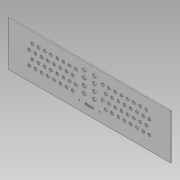
# Autodesk Inventor part: FrontPanel
Saved by Autodesk Inventor 2021.4 (Build 254397000, 397)
## iProperties
Created: 2022-05-18
Part Number: FrontPanel
Material: Generic
Document SubType Name: Modeling
Designer: LaborAdmin
Density: 1 g/cm^3
Appearance: Default
Author: LaborAdmin
Autodesk Inventor part; units mm, degrees
ref_plane "YZ Plane" through (0, 0, 0) normal (1, 0, 0) x (0, 1, 0)
ref_plane "XZ Plane" through (0, 0, 0) normal (0, 1, 0) x (-1, 0, 0)
ref_plane "XY Plane" through (0, 0, 0) normal (0, 0, 1) x (1, 0, 0)
sketch "Sketch1" plane through (0, 0, 0) normal (0, 0, 1) x (1, 0, 0)
  line L0 (-241, 66.5) -> (241, 66.5)
  line L1 (241, 66.5) -> (241, -66.5)
  line L2 (241, -66.5) -> (-241, -66.5)
  line L3 (-241, -66.5) -> (-241, 66.5)
  line L4 (-241, 66.5) -> (241, -66.5) construction
  line L5 (241, 66.5) -> (-241, -66.5) construction
  point P0 (0, 0)
  dimension "d0" = 482
  dimension "d1" = 133
  constraints: 12 end point, 2 midpoint, 2 parallel, 1 horizontal, 1 perpendicular
  measures "d0" distance of L1.end L2.end
  measures "d1" distance of L2.end L0.start
extrude "Extrusion1" add sketch "Sketch1" against normal blind 3
sketch "Sketch2" plane through (0, 0, 0) normal (0, 0, 1) x (1, 0, 0)
  line L0 (-197, -50) -> (197, -50) construction
  line L1 (197, -50) -> (197, 50) construction
  line L2 (197, 50) -> (-197, 50) construction
  line L3 (-197, 50) -> (-197, -50) construction
  line L4 (-197, -50) -> (197, 50) construction
  line L5 (197, -50) -> (-197, 50) construction
  line L6 (-241, 66.5) -> (241, 66.5) construction
  line L7 (0, 66.5) -> (0, -66.5) construction
  line L8 (241, -66.5) -> (-241, -66.5) construction
  line L9 (15, 66.5) -> (15, -66.5) construction
  arc A0 (11.9308, 48.89) -> (18.0692, 48.89) centre (15, 45) ccw
  line L10 (11.9308, 48.89) -> (18.0692, 48.89)
  arc A1 (11.9308, 28.89) -> (18.0692, 28.89) centre (15, 25) ccw
  line L11 (11.9308, 28.89) -> (18.0692, 28.89)
  arc A2 (11.9308, 8.89) -> (18.0692, 8.89) centre (15, 5) ccw
  line L12 (11.9308, 8.89) -> (18.0692, 8.89)
  arc A3 (11.9308, -11.11) -> (18.0692, -11.11) centre (15, -15) ccw
  line L13 (11.9308, -11.11) -> (18.0692, -11.11)
  arc A4 (-18.0692, 48.89) -> (-11.9308, 48.89) centre (-15, 45) ccw
  line L14 (-11.9308, 48.89) -> (-18.0692, 48.89)
  line L15 (-11.9308, 28.89) -> (-18.0692, 28.89)
  arc A5 (-18.0692, 28.89) -> (-11.9308, 28.89) centre (-15, 25) ccw
  line L16 (-11.9308, 8.89) -> (-18.0692, 8.89)
  arc A6 (-18.0692, 8.89) -> (-11.9308, 8.89) centre (-15, 5) ccw
  line L17 (-11.9308, -11.11) -> (-18.0692, -11.11)
  arc A7 (-18.0692, -11.11) -> (-11.9308, -11.11) centre (-15, -15) ccw
  point P0 (0, 0)
  dimension "d4" = 394
  dimension "d5" = 100
  dimension "d6" = 15
  dimension "d7" = 5
  dimension "dBNC" = 9.91
  dimension "hBNC" = 3.89
  dimension "d12" = 9.91
  dimension "d13" = 3.89
  dimension "d14" = 9.91
  dimension "d15" = 3.89
  dimension "d16" = 9.91
  dimension "d17" = 3.89
  dimension "distBNC" = 20
  dimension "d19" = 20
  dimension "d20" = 20
  constraints: 32 end point, 16 point on circle, 16 symmetric about line, 8 centre point, 8 coincident, 6 point on line, 5 horizontal, 4 midpoint, 2 parallel, 1 perpendicular, 1 vertical, 4 other
  measures "d4" distance of L1.end L2.end
  measures "d5" distance of L0.end L1.end
  measures "d6" distance between parallel lines of L7 L9
  measures "d7" distance from line of L2 point (15, 45)
  measures "dBNC" diameter of A0
  measures "hBNC" distance from line of L10 point (15, 45)
  measures "d12" diameter of A1
  measures "d13" distance from line of L11 point (15, 25)
  measures "d14" diameter of A2
  measures "d15" distance from line of L12 point (15, 5)
  measures "d16" diameter of A3
  measures "d17" distance from line of L13 point (15, -15)
  measures "distBNC" distance of point (15, 25) point (15, 45)
  measures "d19" distance of point (15, 5) A1.centre
  measures "d20" distance of point (15, -15) point (15, 5)
extrude "Extrusion2" cut sketch "Sketch2" against normal blind 3
sketch "Sketch3" plane through (0, 0, 0) normal (0, 0, 1) x (1, 0, 0)
  line L0 (-241, 66.5) -> (241, 66.5) projected
  line L1 (0, 66.5) -> (0, -66.5) construction
  line L2 (241, -66.5) -> (-241, -66.5) projected
  line L3 (-197, -50) -> (197, -50) construction
  line L4 (197, -50) -> (197, 50) construction
  line L5 (197, 50) -> (-197, 50) construction
  line L6 (-197, 50) -> (-197, -50) construction
  line L7 (-197, -50) -> (197, 50) construction
  line L8 (197, -50) -> (-197, 50) construction
  arc A0 (11.9308, 48.89) -> (18.0692, 48.89) centre (15, 45) ccw projected
  arc A1 (11.9308, 28.89) -> (18.0692, 28.89) centre (15, 25) ccw projected
  line L9 (15, 45) -> (15, 25) construction
  line L10 (15, 35) -> (197, 35) construction
  arc A2 (11.9308, 8.89) -> (18.0692, 8.89) centre (15, 5) ccw projected
  line L11 (15, 25) -> (15, 5) construction
  arc A3 (11.9308, -11.11) -> (18.0692, -11.11) centre (15, -15) ccw projected
  line L12 (15, 5) -> (15, -15) construction
  line L13 (15, 15) -> (197, 15) construction
  line L14 (15, -5) -> (197, -5) construction
  line L15 (15, -15) -> (15, -35) construction
  line L16 (15, -25) -> (197, -25) construction
  arc A4 (37.5917, 38.225) -> (42.4083, 38.225) centre (40, 35) ccw
  line L17 (37.5917, 38.225) -> (42.4083, 38.225)
  arc A5 (56.0917, 38.225) -> (60.9083, 38.225) centre (58.5, 35) ccw
  line L18 (56.0917, 38.225) -> (60.9083, 38.225)
  arc A6 (74.5917, 38.225) -> (79.4083, 38.225) centre (77, 35) ccw
  line L19 (74.5917, 38.225) -> (79.4083, 38.225)
  arc A7 (93.0917, 38.225) -> (97.9083, 38.225) centre (95.5, 35) ccw
  line L20 (93.0917, 38.225) -> (97.9083, 38.225)
  arc A8 (111.5917, 38.225) -> (116.4083, 38.225) centre (114, 35) ccw
  line L21 (111.5917, 38.225) -> (116.4083, 38.225)
  arc A9 (130.0917, 38.225) -> (134.9083, 38.225) centre (132.5, 35) ccw
  line L22 (130.0917, 38.225) -> (134.9083, 38.225)
  arc A10 (148.5917, 38.225) -> (153.4083, 38.225) centre (151, 35) ccw
  line L23 (148.5917, 38.225) -> (153.4083, 38.225)
  arc A11 (167.0917, 38.225) -> (171.9083, 38.225) centre (169.5, 35) ccw
  line L24 (167.0917, 38.225) -> (171.9083, 38.225)
  arc A12 (46.8417, 18.225) -> (51.6583, 18.225) centre (49.25, 15) ccw
  line L25 (46.8417, 18.225) -> (51.6583, 18.225)
  arc A13 (65.3417, 18.225) -> (70.1583, 18.225) centre (67.75, 15) ccw
  line L26 (65.3417, 18.225) -> (70.1583, 18.225)
  arc A14 (83.8417, 18.225) -> (88.6583, 18.225) centre (86.25, 15) ccw
  line L27 (83.8417, 18.225) -> (88.6583, 18.225)
  arc A15 (102.3417, 18.225) -> (107.1583, 18.225) centre (104.75, 15) ccw
  line L28 (102.3417, 18.225) -> (107.1583, 18.225)
  arc A16 (120.8417, 18.225) -> (125.6583, 18.225) centre (123.25, 15) ccw
  line L29 (120.8417, 18.225) -> (125.6583, 18.225)
  arc A17 (139.3417, 18.225) -> (144.1583, 18.225) centre (141.75, 15) ccw
  line L30 (139.3417, 18.225) -> (144.1583, 18.225)
  arc A18 (157.8417, 18.225) -> (162.6583, 18.225) centre (160.25, 15) ccw
  line L31 (157.8417, 18.225) -> (162.6583, 18.225)
  arc A19 (176.3417, 18.225) -> (181.1583, 18.225) centre (178.75, 15) ccw
  line L32 (176.3417, 18.225) -> (181.1583, 18.225)
  arc A20 (37.5917, -1.775) -> (42.4083, -1.775) centre (40, -5) ccw
  line L33 (37.5917, -1.775) -> (42.4083, -1.775)
  line L34 (56.0917, -1.775) -> (60.9083, -1.775)
  arc A21 (56.0917, -1.775) -> (60.9083, -1.775) centre (58.5, -5) ccw
  line L35 (74.5917, -1.775) -> (79.4083, -1.775)
  arc A22 (74.5917, -1.775) -> (79.4083, -1.775) centre (77, -5) ccw
  line L36 (93.0917, -1.775) -> (97.9083, -1.775)
  arc A23 (93.0917, -1.775) -> (97.9083, -1.775) centre (95.5, -5) ccw
  line L37 (111.5917, -1.775) -> (116.4083, -1.775)
  arc A24 (111.5917, -1.775) -> (116.4083, -1.775) centre (114, -5) ccw
  line L38 (130.0917, -1.775) -> (134.9083, -1.775)
  arc A25 (130.0917, -1.775) -> (134.9083, -1.775) centre (132.5, -5) ccw
  line L39 (148.5917, -1.775) -> (153.4083, -1.775)
  arc A26 (148.5917, -1.775) -> (153.4083, -1.775) centre (151, -5) ccw
  line L40 (167.0917, -1.775) -> (171.9083, -1.775)
  arc A27 (167.0917, -1.775) -> (171.9083, -1.775) centre (169.5, -5) ccw
  arc A28 (46.8417, -21.775) -> (51.6583, -21.775) centre (49.25, -25) ccw
  line L41 (46.8417, -21.775) -> (51.6583, -21.775)
  arc A29 (65.3417, -21.775) -> (70.1583, -21.775) centre (67.75, -25) ccw
  line L42 (65.3417, -21.775) -> (70.1583, -21.775)
  arc A30 (83.8417, -21.775) -> (88.6583, -21.775) centre (86.25, -25) ccw
  line L43 (83.8417, -21.775) -> (88.6583, -21.775)
  arc A31 (102.3417, -21.775) -> (107.1583, -21.775) centre (104.75, -25) ccw
  line L44 (102.3417, -21.775) -> (107.1583, -21.775)
  arc A32 (120.8417, -21.775) -> (125.6583, -21.775) centre (123.25, -25) ccw
  line L45 (120.8417, -21.775) -> (125.6583, -21.775)
  arc A33 (139.3417, -21.775) -> (144.1583, -21.775) centre (141.75, -25) ccw
  line L46 (139.3417, -21.775) -> (144.1583, -21.775)
  arc A34 (157.8417, -21.775) -> (162.6583, -21.775) centre (160.25, -25) ccw
  line L47 (157.8417, -21.775) -> (162.6583, -21.775)
  arc A35 (176.3417, -21.775) -> (181.1583, -21.775) centre (178.75, -25) ccw
  line L48 (176.3417, -21.775) -> (181.1583, -21.775)
  arc A36 (-42.4083, 38.225) -> (-37.5917, 38.225) centre (-40, 35) ccw
  line L49 (-37.5917, 38.225) -> (-42.4083, 38.225)
  line L50 (-56.0917, 38.225) -> (-60.9083, 38.225)
  arc A37 (-60.9083, 38.225) -> (-56.0917, 38.225) centre (-58.5, 35) ccw
  line L51 (-74.5917, 38.225) -> (-79.4083, 38.225)
  arc A38 (-79.4083, 38.225) -> (-74.5917, 38.225) centre (-77, 35) ccw
  line L52 (-93.0917, 38.225) -> (-97.9083, 38.225)
  arc A39 (-97.9083, 38.225) -> (-93.0917, 38.225) centre (-95.5, 35) ccw
  line L53 (-111.5917, 38.225) -> (-116.4083, 38.225)
  arc A40 (-116.4083, 38.225) -> (-111.5917, 38.225) centre (-114, 35) ccw
  line L54 (-130.0917, 38.225) -> (-134.9083, 38.225)
  arc A41 (-134.9083, 38.225) -> (-130.0917, 38.225) centre (-132.5, 35) ccw
  line L55 (-148.5917, 38.225) -> (-153.4083, 38.225)
  arc A42 (-153.4083, 38.225) -> (-148.5917, 38.225) centre (-151, 35) ccw
  line L56 (-167.0917, 38.225) -> (-171.9083, 38.225)
  arc A43 (-171.9083, 38.225) -> (-167.0917, 38.225) centre (-169.5, 35) ccw
  arc A44 (-51.6583, 18.225) -> (-46.8417, 18.225) centre (-49.25, 15) ccw
  line L57 (-46.8417, 18.225) -> (-51.6583, 18.225)
  arc A45 (-70.1583, 18.225) -> (-65.3417, 18.225) centre (-67.75, 15) ccw
  line L58 (-65.3417, 18.225) -> (-70.1583, 18.225)
  arc A46 (-88.6583, 18.225) -> (-83.8417, 18.225) centre (-86.25, 15) ccw
  line L59 (-83.8417, 18.225) -> (-88.6583, 18.225)
  arc A47 (-107.1583, 18.225) -> (-102.3417, 18.225) centre (-104.75, 15) ccw
  line L60 (-102.3417, 18.225) -> (-107.1583, 18.225)
  arc A48 (-125.6583, 18.225) -> (-120.8417, 18.225) centre (-123.25, 15) ccw
  line L61 (-120.8417, 18.225) -> (-125.6583, 18.225)
  arc A49 (-144.1583, 18.225) -> (-139.3417, 18.225) centre (-141.75, 15) ccw
  line L62 (-139.3417, 18.225) -> (-144.1583, 18.225)
  arc A50 (-162.6583, 18.225) -> (-157.8417, 18.225) centre (-160.25, 15) ccw
  line L63 (-157.8417, 18.225) -> (-162.6583, 18.225)
  arc A51 (-181.1583, 18.225) -> (-176.3417, 18.225) centre (-178.75, 15) ccw
  line L64 (-176.3417, 18.225) -> (-181.1583, 18.225)
  arc A52 (-42.4083, -1.775) -> (-37.5917, -1.775) centre (-40, -5) ccw
  line L65 (-74.5917, -1.775) -> (-79.4083, -1.775)
  line L66 (-83.8417, -21.775) -> (-88.6583, -21.775)
  line L67 (-65.3417, -21.775) -> (-70.1583, -21.775)
  arc A53 (-70.1583, -21.775) -> (-65.3417, -21.775) centre (-67.75, -25) ccw
  arc A54 (-88.6583, -21.775) -> (-83.8417, -21.775) centre (-86.25, -25) ccw
  line L68 (-102.3417, -21.775) -> (-107.1583, -21.775)
  arc A55 (-107.1583, -21.775) -> (-102.3417, -21.775) centre (-104.75, -25) ccw
  line L69 (-56.0917, -1.775) -> (-60.9083, -1.775)
  arc A56 (-60.9083, -1.775) -> (-56.0917, -1.775) centre (-58.5, -5) ccw
  arc A57 (-79.4083, -1.775) -> (-74.5917, -1.775) centre (-77, -5) ccw
  line L70 (-93.0917, -1.775) -> (-97.9083, -1.775)
  arc A58 (-97.9083, -1.775) -> (-93.0917, -1.775) centre (-95.5, -5) ccw
  line L71 (-130.0917, -1.775) -> (-134.9083, -1.775)
  arc A59 (-134.9083, -1.775) -> (-130.0917, -1.775) centre (-132.5, -5) ccw
  line L72 (-120.8417, -21.775) -> (-125.6583, -21.775)
  arc A60 (-125.6583, -21.775) -> (-120.8417, -21.775) centre (-123.25, -25) ccw
  line L73 (-111.5917, -1.775) -> (-116.4083, -1.775)
  arc A61 (-116.4083, -1.775) -> (-111.5917, -1.775) centre (-114, -5) ccw
  line L74 (-176.3417, -21.775) -> (-181.1583, -21.775)
  arc A62 (-181.1583, -21.775) -> (-176.3417, -21.775) centre (-178.75, -25) ccw
  arc A63 (-144.1583, -21.775) -> (-139.3417, -21.775) centre (-141.75, -25) ccw
  line L75 (-139.3417, -21.775) -> (-144.1583, -21.775)
  line L76 (-148.5917, -1.775) -> (-153.4083, -1.775)
  arc A64 (-153.4083, -1.775) -> (-148.5917, -1.775) centre (-151, -5) ccw
  arc A65 (-162.6583, -21.775) -> (-157.8417, -21.775) centre (-160.25, -25) ccw
  line L77 (-157.8417, -21.775) -> (-162.6583, -21.775)
  arc A66 (-171.9083, -1.775) -> (-167.0917, -1.775) centre (-169.5, -5) ccw
  line L78 (-167.0917, -1.775) -> (-171.9083, -1.775)
  line L79 (-37.5917, -1.775) -> (-42.4083, -1.775)
  line L80 (-46.8417, -21.775) -> (-51.6583, -21.775)
  arc A67 (-51.6583, -21.775) -> (-46.8417, -21.775) centre (-49.25, -25) ccw
  point P0 (0, 0)
  dimension "d23" = 394
  dimension "d24" = 100
  dimension "d25" = 20
  dimension "dXLR" = 8.05
  dimension "distBNC_XLR" = 25
  dimension "hXLR" = 7.25
  dimension "d29" = 8.05
  dimension "d30" = 7.25
  dimension "d31" = 8.05
  dimension "d32" = 7.25
  dimension "d33" = 8.05
  dimension "d34" = 7.25
  dimension "d35" = 8.05
  dimension "d36" = 7.25
  dimension "d37" = 8.05
  dimension "d38" = 7.25
  dimension "d39" = 8.05
  dimension "d40" = 7.25
  dimension "d41" = 8.05
  dimension "d42" = 7.25
  dimension "distXLR" = 18.5
  dimension "d44" = 18.5
  dimension "d45" = 18.5
  dimension "d46" = 18.5
  dimension "d47" = 18.5
  dimension "d48" = 18.5
  dimension "d49" = 18.5
  dimension "d50" = 8.05
  dimension "d73" = 34.25
  dimension "d74" = 7.25
  dimension "d75" = 8.05
  dimension "d76" = 7.25
  dimension "d77" = 8.05
  dimension "d78" = 7.25
  dimension "d79" = 8.05
  dimension "d80" = 7.25
  dimension "d81" = 8.05
  dimension "d82" = 7.25
  dimension "d83" = 8.05
  dimension "d84" = 7.25
  dimension "d85" = 8.05
  dimension "d86" = 7.25
  dimension "d87" = 8.05
  dimension "d88" = 7.25
  dimension "d89" = 18.5
  dimension "d90" = 18.5
  dimension "d91" = 18.5
  dimension "d92" = 18.5
  dimension "d93" = 18.5
  dimension "d94" = 18.5
  dimension "d95" = 18.5
  dimension "d96" = 8.05
  dimension "d98" = 8.05
  dimension "d100" = 8.05
  dimension "d102" = 8.05
  dimension "d104" = 8.05
  dimension "d106" = 8.05
  dimension "d108" = 8.05
  dimension "d110" = 8.05
  dimension "d112" = 18.5
  dimension "d113" = 18.5
  dimension "d114" = 18.5
  dimension "d115" = 18.5
  dimension "d116" = 18.5
  constraints: 150 end point, 128 point on circle, 96 symmetric about line, 64 centre point, 33 horizontal, 8 midpoint, 8 vertical, 4 point on line, 2 parallel, 1 perpendicular, 76 other
  measures "d23" distance of L4.end L5.end
  measures "d24" distance of L3.end L4.end
  measures "d25" distance of L12.end L15.end
  measures "dXLR" diameter of A4
  measures "distBNC_XLR" distance of A4.centre point (15, 35)
  measures "d29" diameter of A5
  measures "d31" diameter of A6
  measures "d33" diameter of A7
  measures "d35" diameter of A8
  measures "d37" diameter of A9
  measures "d39" diameter of A10
  measures "d41" diameter of A11
  measures "distXLR" distance of A5.centre A4.centre
  measures "d44" distance of A6.centre A5.centre
  measures "d45" distance of A7.centre A6.centre
  measures "d46" distance of A8.centre A7.centre
  measures "d47" distance of A9.centre A8.centre
  measures "d48" distance of A11.centre A10.centre
  measures "d49" distance of A10.centre A9.centre
  measures "d50" diameter of A12
  measures "d73" distance of A12.centre point (15, 15)
  measures "d75" diameter of A13
  measures "d77" diameter of A14
  measures "d79" diameter of A15
  measures "d81" diameter of A16
  measures "d83" diameter of A17
  measures "d85" diameter of A18
  measures "d87" diameter of A19
  measures "d89" distance of A13.centre A12.centre
  measures "d90" distance of A14.centre A13.centre
  measures "d91" distance of A15.centre A14.centre
  measures "d92" distance of A16.centre A15.centre
  measures "d93" distance of A17.centre A16.centre
  measures "d94" distance of A18.centre A17.centre
  measures "d95" distance of A19.centre A18.centre
  measures "d96" diameter of A20
  measures "d98" diameter of A21
  measures "d100" diameter of A22
  measures "d102" diameter of A23
  measures "d104" diameter of A24
  measures "d106" diameter of A25
  measures "d108" diameter of A26
  measures "d110" diameter of A27
  measures "d112" distance of A21.centre A20.centre
  measures "d113" distance of A22.centre A21.centre
  measures "d114" distance of A23.centre A22.centre
  measures "d115" distance of A24.centre A23.centre
  measures "d116" distance of A25.centre A24.centre
extrude "Extrusion3" cut sketch "Sketch3" against normal blind 3
sketch "Sketch4" plane through (0, 0, 0) normal (0, 0, 1) x (1, 0, 0)
  line L0 (-241, 66.5) -> (241, 66.5) projected
  line L1 (0, 66.5) -> (0, -66.5) construction
  line L2 (241, -66.5) -> (-241, -66.5) projected
  line L3 (241, 66.5) -> (-241, 66.5) projected
  line L4 (-241, -66.5) -> (241, -66.5) projected
  line L5 (-11, -42.5) -> (11, -42.5)
  line L6 (12.5, -41) -> (12.5, -39)
  line L7 (11, -37.5) -> (-11, -37.5)
  line L8 (-12.5, -39) -> (-12.5, -41)
  line L9 (-12.5, -42.5) -> (12.5, -37.5) construction
  line L10 (12.5, -42.5) -> (-12.5, -37.5) construction
  circle A0 centre (0, -40) radius 15 construction
  circle A1 centre (30, -40) radius 1.5
  line L11 (0, -40) -> (30, -40) construction
  circle A2 centre (-30, -40) radius 1.5
  arc A3 (-11, -37.5) -> (-12.5, -39) centre (-11, -39) ccw
  arc A4 (-12.5, -41) -> (-11, -42.5) centre (-11, -41) ccw
  arc A5 (12.5, -39) -> (11, -37.5) centre (11, -39) ccw
  arc A6 (11, -42.5) -> (12.5, -41) centre (11, -41) ccw
  point P0 (0, 0)
  point P1 (0, 66.5)
  dimension "d162" = 25
  dimension "d163" = 5
  dimension "d164" = 40
  dimension "d165" = 30
  dimension "d166" = 3
  dimension "d167" = 17.5
  dimension "d170" = 1.5
  constraints: 16 end point, 9 point on line, 8 midpoint, 8 point on circle, 8 tangent, 7 centre point, 3 equal radius, 2 horizontal, 2 parallel, 1 coincident, 1 perpendicular, 1 symmetric about line, 1 other
  measures "d162" distance of L9.end L10.end
  measures "d163" distance of L10.start L9.end
  measures "d164" distance of point (0, -40) point (0, 0)
  measures "d165" diameter of A0
  measures "d166" diameter of A1
  measures "d167" distance from line of L11.end L6
  measures "d170" radius of A3
extrude "Extrusion4" cut sketch "Sketch4" against normal blind 3
equation "\"d12\" = dBNC"
equation "\"d13\" = hBNC"
equation "\"d14\" = dBNC"
equation "\"d15\" = hBNC"
equation "\"d16\" = dBNC"
equation "\"d17\" = hBNC"
equation "\"d19\" = distBNC"
equation "\"d20\" = distBNC"
equation "\"d25\" = distBNC"
equation "\"d44\" = distXLR"
equation "\"d45\" = distXLR"
equation "\"d46\" = distXLR"
equation "\"d47\" = distXLR"
equation "\"d48\" = distXLR"
equation "\"d49\" = distXLR"
equation "\"d89\" = distXLR"
equation "\"d90\" = distXLR"
body "Solid1"
